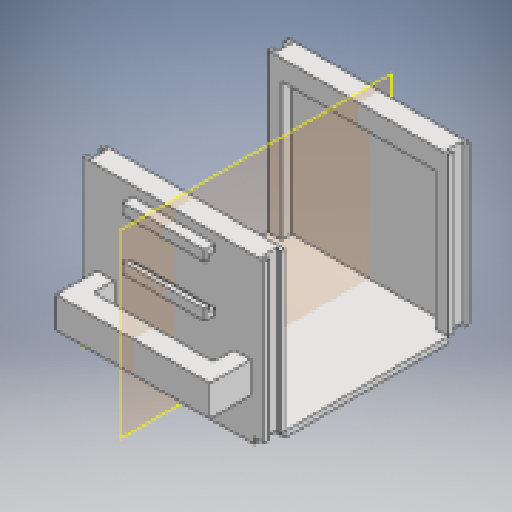
# Autodesk Inventor part: maindrawer
Saved by Autodesk Inventor 2025.2 (Build 292293000, 293)
## iProperties
Created: 2025-02-24
Part Number: maindrawer
Material: Generic
Document SubType Name: Modeling
Designer: email
Density: 1 g/cm^3
Appearance: Default
Author: email
Autodesk Inventor part; units mm, degrees
ref_plane "YZ Plane" through (0, 0, 0) normal (1, 0, 0) x (0, 1, 0)
ref_plane "XZ Plane" through (0, 0, 0) normal (0, 1, 0) x (-1, 0, 0)
ref_plane "XY Plane" through (0, 0, 0) normal (0, 0, 1) x (1, 0, 0)
sketch "Sketch1" plane through (0, 0, 0) normal (0, 1, 0) x (-1, 0, 0)
  line L0 (0, 0) -> (-88, 0)
  line L1 (-88, 0) -> (-88, -90)
  line L2 (-88, -90) -> (0, -90)
  line L3 (0, -90) -> (0, 0)
  line L4 (0, -90) -> (-88, -90)
  line L5 (-88, -90) -> (-88, -80)
  line L6 (-88, -80) -> (0, -80)
  line L7 (0, -80) -> (0, -90)
  line L8 (0, 0) -> (-88, 0)
  line L9 (-88, 0) -> (-88, 10)
  line L10 (-88, 10) -> (0, 10)
  line L11 (0, 10) -> (0, 0)
  point P0 (0, -80)
  dimension "d0" = 88
  dimension "d1" = 90
  dimension "d2" = 10
  dimension "d3" = 10
  constraints: 24 end point, 6 parallel, 3 horizontal, 3 perpendicular, 1 collinear, 1 point on line
  measures "d0" distance between parallel lines of L1 L3
  measures "d1" distance between parallel lines of L0 L2
  measures "d2" distance between parallel lines of L2 L6
  measures "d3" distance of L10.end L0.start
extrude "Extrusion1" add sketch "Sketch1" along normal blind 3
extrude "Extrusion2" add sketch "Sketch1" along normal blind 80 contours L0 L9 L10 L11 | L3 L2 L1 L6
sketch "Sketch2" plane through (0, 80, 0) normal (0, 1, 0) x (1, 0, 0)
  line L0 (0, 90) -> (0, 80) projected
  line L1 (0, 87.5) -> (2.5, 89)
  line L2 (2.5, 89) -> (2.5, 81)
  line L3 (2.5, 81) -> (0, 82.5)
  line L4 (0, 87.5) -> (0, 82.5)
  line L5 (88, 90) -> (0, 90) projected
  line L6 (44, 90) -> (44, -10) construction
  line L7 (0, -10) -> (88, -10) projected
  line L8 (88, 90) -> (88, 80)
  line L9 (88, 87.5) -> (85.5, 89)
  line L10 (85.5, 89) -> (85.5, 81)
  line L11 (85.5, 81) -> (88, 82.5)
  line L12 (88, 87.5) -> (88, 82.5)
  line L13 (0, 0) -> (0, -10) projected
  line L14 (0, -2.5) -> (2.5, -1)
  line L15 (2.5, -1) -> (2.5, -9)
  line L16 (2.5, -9) -> (0, -7.5)
  line L17 (0, -7.5) -> (0, -2.5)
  line L18 (88, -10) -> (0, -10)
  line L19 (88, 0) -> (88, -10)
  line L20 (88, -2.5) -> (85.5, -1)
  line L21 (85.5, -1) -> (85.5, -9)
  line L22 (85.5, -9) -> (88, -7.5)
  line L23 (88, -7.5) -> (88, -2.5)
  point P0 (2.5, 85)
  point P1 (0, 85)
  point P2 (0, 85)
  point P3 (85.5, 85)
  point P4 (88, 85)
  point P5 (88, 85)
  point P6 (12.8674, 46.7636)
  point P7 (2.5, -5)
  point P8 (0, -5)
  point P9 (0, -5)
  point P10 (85.5, -5)
  point P11 (88, -5)
  point P12 (88, -5)
  dimension "d11" = 8
  dimension "d12" = 5
  dimension "d13" = 2.5
  dimension "d14" = 5
  dimension "d19" = 8
  dimension "d20" = 5
  dimension "d21" = 2.5
  constraints: 40 end point, 18 symmetric about line, 9 midpoint, 8 point on line, 2 collinear, 2 horizontal alignment, 2 parallel, 1 coincident
  measures "d11" distance of L1.end L2.end
  measures "d12" distance of L3.end L1.start
  measures "d13" distance between parallel lines of L0 L2
  measures "d14" distance from line of L5 point (0, 85)
  measures "d19" distance of L14.end L15.end
  measures "d20" distance of L16.end L14.start
  measures "d21" distance between parallel lines of L15 L17
extrude "Extrusion3" cut sketch "Sketch2" against normal blind 88
sketch "Sketch3" plane through (0, 0, 0) normal (0, -1, 0) x (1, 0, 0)
  line L0 (0, 10) -> (88, 10) projected
  line L1 (88, 0) -> (0, 0) projected
  line L2 (0, 10) -> (5, 10)
  line L3 (5, 10) -> (5, 0)
  line L4 (5, 0) -> (0, 0)
  line L5 (0, 0) -> (0, 10)
  line L6 (88, 10) -> (83, 10)
  line L7 (83, 10) -> (83, 0)
  line L8 (83, 0) -> (88, 0)
  line L9 (88, 0) -> (88, 10)
  line L10 (88, 10) -> (88, 7.5) projected
  line L11 (88, -80) -> (0, -80) projected
  line L12 (88, -90) -> (0, -90) projected
  line L13 (0, -80) -> (5, -80)
  line L14 (5, -80) -> (5, -90)
  line L15 (5, -90) -> (0, -90)
  line L16 (0, -90) -> (0, -80)
  line L17 (88, -80) -> (83, -80)
  line L18 (83, -80) -> (83, -90)
  line L19 (83, -90) -> (88, -90)
  line L20 (88, -90) -> (88, -80)
  point P0 (88, 8.75)
  point P1 (0, -90)
  point P2 (5, -80)
  point P3 (88, -80)
  point P4 (83, -80)
  point P5 (5, 10)
  dimension "d24" = 5
  dimension "d25" = 5
  dimension "d26" = 5
  dimension "d27" = 5
  constraints: 32 end point, 8 parallel, 5 point on line, 4 horizontal, 4 perpendicular, 1 midpoint
  measures "d24" distance between parallel lines of L5 L3
  measures "d25" distance from line of point (88, 8.75) L7
  measures "d26" distance between parallel lines of L16 L14
  measures "d27" distance between parallel lines of L20 L18
extrude "Extrusion4" cut sketch "Sketch3" against normal blind 3 contours L0 L3 L1 L5 | L0 L9 L1 L7 | L20 L12 L18 L11 | L14 L12 L16 L11
ref_plane "Work Plane1" through (0, 70, 0) normal (0, 1, 0) x (1, 0, 0)
sketch "Sketch4" plane through (0, 70, 0) normal (0, 1, 0) x (1, 0, 0)
  line L0 (0, 80) -> (88, 80) projected
  line L1 (6.5, 85) -> (81.5, 85)
  line L2 (81.5, 85) -> (81.5, 80)
  line L3 (81.5, 80) -> (6.5, 80)
  line L4 (6.5, 80) -> (6.5, 85)
  line L5 (0, 82.5) -> (0, 80) projected
  line L6 (10.5, 0) -> (77.5, 0)
  line L7 (77.5, 0) -> (77.5, -5)
  line L8 (77.5, -5) -> (10.5, -5)
  line L9 (10.5, -5) -> (10.5, 0)
  line L10 (5, 0) -> (83, 0) projected
  point P0 (0, 0)
  point P1 (44, 85)
  point P2 (44, 80)
  point P3 (44, 80)
  point P4 (44, -5)
  dimension "d31" = 5
  dimension "d32" = 75
  dimension "d34" = 5
  constraints: 16 end point, 4 midpoint, 4 parallel, 2 horizontal, 2 perpendicular, 2 vertical alignment, 1 coincident, 1 collinear, 1 point on line
  measures "d31" distance between parallel lines of L0 L1
  measures "d32" distance between parallel lines of L2 L4
  measures "d34" distance between parallel lines of L6 L8
extrude "Extrusion5" cut sketch "Sketch4" against normal up to surface (67 mm away)
sketch "Sketch5" plane through (0, 80, 10) normal (0, 0, 1) x (1, 0, 0)
  point P0 (0, -80)
sketch "Sketch6" plane through (0, 80, 10) normal (0, 0, 1) x (1, 0, 0)
  line L0 (24, -5) -> (64, -5)
  line L1 (64, -5) -> (64, -10)
  line L2 (64, -10) -> (24, -10)
  line L3 (24, -10) -> (24, -5)
  line L4 (24, -30) -> (64, -30)
  line L5 (64, -30) -> (64, -35)
  line L6 (64, -35) -> (24, -35)
  line L7 (24, -35) -> (24, -30)
  line L8 (0, 0) -> (88, 0) projected
  line L9 (6.5, -45) -> (81.5, -45)
  line L10 (81.5, -45) -> (81.5, -60)
  line L11 (81.5, -60) -> (6.5, -60)
  line L12 (6.5, -60) -> (6.5, -45)
  line L13 (5, -80) -> (83, -80) projected
  point P0 (0, -80)
  point P1 (44, -5)
  point P2 (44, 0)
  point P3 (44, -45)
  point P4 (44, 0)
  dimension "d37" = 40
  dimension "d38" = 5
  dimension "d39" = 5
  dimension "d40" = 20
  dimension "d41" = 5
  dimension "d42" = 15
  dimension "d43" = 75
  dimension "d44" = 20
  constraints: 24 end point, 6 parallel, 4 midpoint, 3 horizontal, 3 perpendicular, 2 point on line, 2 vertical alignment
  measures "d37" distance between parallel lines of L1 L3
  measures "d38" distance between parallel lines of L2 L0
  measures "d39" distance between parallel lines of L6 L4
  measures "d40" distance between parallel lines of L4 L2
  measures "d41" distance between parallel lines of L8 L0
  measures "d42" distance between parallel lines of L11 L9
  measures "d43" distance between parallel lines of L10 L12
  measures "d44" distance between parallel lines of L13 L11
extrude "Extrusion6" add sketch "Sketch6" along normal blind 5 contours L0 L1 L2 L3 | L4 L5 L6 L7
extrude "Extrusion7" add sketch "Sketch6" along normal blind 20 contours L9 L10 L11 L12
sketch "Sketch7" plane through (6.5, 35, 10) normal (0, 1, 0) x (1, 0, 0)
  line L0 (-1.5, 0) -> (76.5, 0) projected
  line L1 (8.3358, 0) -> (66.6642, 0)
  line L2 (66.6642, 0) -> (66.6642, -10)
  line L3 (66.6642, -10) -> (8.3358, -10)
  line L4 (8.3358, -10) -> (8.3358, 0)
  line L5 (-6.5, 0) -> (81.5, 0) projected
  point P0 (-6.5, 10)
  point P1 (37.5, -10)
  point P2 (37.5, 0)
  point P3 (66.6642, 0)
  dimension "d49" = 10
  constraints: 8 end point, 2 midpoint, 2 parallel, 1 horizontal, 1 perpendicular, 1 point on line, 1 vertical alignment
  measures "d49" distance of L3.end L1.start
extrude "Extrusion8" cut sketch "Sketch7" against normal up to surface (15 mm away)
sketch "Sketch8" plane through (64, 70, 10) normal (1, 0, 0) x (0, 0, -1)
  line L0 (0, 0) -> (-5, 0) projected
  line L1 (0, 0) -> (-2.689, 0)
  line L2 (-2.689, 0) -> (-2.689, 2)
  line L3 (-2.689, 2) -> (0, 2)
  line L4 (0, 2) -> (0, 0)
  line L5 (0, -20) -> (-5, -20) projected
  line L6 (0, -20) -> (-2.689, -20)
  line L7 (-2.689, -20) -> (-2.689, -22)
  line L8 (-2.689, -22) -> (0, -22)
  line L9 (0, -22) -> (0, -20)
  point P0 (10, -70)
  point P1 (-2.5, 0)
  point P2 (-2.5, -20)
  point P3 (-2.689, -20)
  dimension "d52" = 2
  dimension "d53" = 2
  constraints: 16 end point, 4 parallel, 2 horizontal, 2 midpoint, 2 perpendicular, 1 collinear
  measures "d52" distance from line of point (-2.5, 0) L3
  measures "d53" distance from line of point (-2.5, -20) L8
extrude "Extrusion9" cut sketch "Sketch8" against normal up to surface (40 mm away)
sketch "Sketch9" plane through (0, 80, 7.5) normal (-1, 0, 0) x (0, 0, 1)
  line L0 (2.5, -77) -> (2.5, -80) projected
  line L1 (-97.5, 0) -> (2.5, 0)
  line L2 (2.5, 0) -> (2.5, -80)
  line L3 (2.5, -80) -> (-97.5, -80)
  line L4 (-97.5, -80) -> (-97.5, 0)
  point P0 (-7.5, -80)
  constraints: 8 end point, 2 parallel, 1 horizontal, 1 perpendicular
extrude "Extrusion10" cut sketch "Sketch9" against normal blind 0.1
ref_plane "Work Plane2" through (44, 45, 15) normal (1, 0, 0) x (0, 0, -1)
mirror "Mirror1" about plane through (44, 45, 15) normal (1, 0, 0) of "Extrusion10"
sketch "Sketch10" plane through (6.5, 70, -80) normal (0, 0, 1) x (1, 0, 0)
  line L0 (81.4, -67) -> (81.4, 10) projected
  line L1 (-6.4, 10) -> (81.4, 10) projected
  line L2 (-6.4, 10) -> (-6.4, -67) projected
  line L3 (-1.5, -67) -> (-6.4, -67) projected
  line L4 (0, -67) -> (-1.5, -67) projected
  line L5 (0, -67) -> (0, 0) projected
  line L6 (0, 0) -> (75, 0) projected
  line L7 (75, 0) -> (75, -67) projected
  line L8 (76.5, -67) -> (75, -67) projected
  line L9 (81.4, -67) -> (76.5, -67) projected
  point P0 (-6.5, -70)
extrude "Extrusion11" add sketch "Sketch10" along normal blind 0.1
sketch "Sketch11" plane through (77.5, 70, 0) normal (0, 0, -1) x (-1, 0, 0)
  line L0 (-10.4, 10) -> (-10.4, -67) projected
  line L1 (-5.5, -67) -> (-10.4, -67) projected
  line L2 (0, -67) -> (-5.5, -67) projected
  line L3 (0, -67) -> (0, 0) projected
  line L4 (0, 0) -> (67, 0) projected
  line L5 (67, 0) -> (67, -67) projected
  line L6 (72.5, -67) -> (67, -67) projected
  line L7 (77.4, -67) -> (72.5, -67) projected
  line L8 (77.4, -67) -> (77.4, 10) projected
  line L9 (-10.4, 10) -> (77.4, 10) projected
  point P0 (77.5, -70)
extrude "Extrusion12" add sketch "Sketch11" along normal blind 0.1
sketch "Sketch12" plane through (0, 80, 0) normal (0, 1, 0) x (1, 0, 0)
  line L0 (87.9, -10) -> (87.9, -7.56) projected
  line L1 (87.9, -7.56) -> (85.5, -9) projected
  line L2 (85.5, -9) -> (85.5, -1) projected
  line L3 (85.5, -1) -> (87.9, -2.44) projected
  line L4 (87.9, -2.44) -> (87.9, 0.1) projected
  line L5 (0.1, 0.1) -> (87.9, 0.1) projected
  line L6 (0.1, -2.44) -> (0.1, 0.1) projected
  line L7 (0.1, -2.44) -> (2.5, -1) projected
  line L8 (2.5, -1) -> (2.5, -9) projected
  line L9 (2.5, -9) -> (0.1, -7.56) projected
  line L10 (0.1, -7.56) -> (0.1, -10) projected
  line L11 (0.1, -10) -> (87.9, -10) projected
  line L12 (87.9, 87.56) -> (87.9, 90) projected
  line L13 (87.9, 90) -> (0.1, 90) projected
  line L14 (0.1, 90) -> (0.1, 87.56) projected
  line L15 (0.1, 87.56) -> (2.5, 89) projected
  line L16 (2.5, 89) -> (2.5, 81) projected
  line L17 (2.5, 81) -> (0.1, 82.44) projected
  line L18 (0.1, 82.44) -> (0.1, 79.9) projected
  line L19 (87.9, 79.9) -> (0.1, 79.9) projected
  line L20 (87.9, 82.44) -> (87.9, 79.9) projected
  line L21 (87.9, 82.44) -> (85.5, 81) projected
  line L22 (85.5, 81) -> (85.5, 89) projected
  line L23 (85.5, 89) -> (87.9, 87.56) projected
  point P0 (0, 0)
extrude "Extrusion13" cut sketch "Sketch12" against normal blind 0.2
sketch "Sketch13" plane through (0, 0, 0) normal (0, -1, 0) x (1, 0, 0)
  line L0 (87.9, -80) -> (87.9, 0) projected
  line L1 (87.9, 0) -> (83, 0) projected
  line L2 (83, 0) -> (83, 10) projected
  line L3 (5, 10) -> (83, 10) projected
  line L4 (5, 10) -> (5, 0) projected
  line L5 (5, 0) -> (0.1, 0) projected
  line L6 (0.1, 0) -> (0.1, -80) projected
  line L7 (0.1, -80) -> (5, -80) projected
  line L8 (5, -80) -> (5, -90) projected
  line L9 (83, -90) -> (5, -90) projected
  line L10 (83, -90) -> (83, -80) projected
  line L11 (83, -80) -> (87.9, -80) projected
  point P0 (0, 0)
extrude "Extrusion14" cut sketch "Sketch13" against normal blind 0.2
equation "\"d22\" = d0"
equation "\"d56\" = tol"
equation "\"d58\" = tol"
equation "\"d62\" = 2 * tol"
equation "\"d64\" = 2 * tol"
equation "\"tol\" = 0.1"
body "Solid1"
